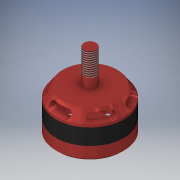
# Autodesk Inventor part: Motor
Saved by Autodesk Inventor 2019.3 (Build 233278000, 278)
## iProperties
Created: 2019-02-12
Part Number: Motor
Material: Aluminum 6061
Document SubType Name: Modeling
Designer: JMoll
Density: 2.7 g/cm^3
Appearance: Aluminum - Polished(1)
Author: JMoll
Autodesk Inventor part; units mm, degrees
sketch "Sketch1" plane through (0, 0, 0) normal (0, 0, 1) x (1, 0, 0)
  line L0 (0, 0) -> (0, 17.2)
  line L1 (0, 17.2) -> (11.25, 17.2)
  line L2 (11.25, 17.2) -> (14, 13.2)
  line L3 (14, 13.2) -> (14, 0)
  line L4 (14, 0) -> (0, 0)
  dimension "d0" = 17.2
  dimension "d1" = 28
  dimension "d2" = 22.5
  dimension "d3" = 13.2
  constraints: 10 end point, 2 perpendicular, 1 parallel, 1 vertical
  measures "d0" distance of L0.start L0.end
  measures "d1" diameter of L3 L0
  measures "d2" diameter of L1.end L0
  measures "d3" distance of L2.end L3.end
revolve "Revolution1" add sketch "Sketch1" angle 360 about axis through (0, 0, 0) along (0, 1, 0)
shell "Shell1" thickness 2.5 removed faces 0 ; own thickness 1 on faces at (1.3298, 17.2, -1.7114) ; own thickness 3.5 on faces at (2.651, 0, -3.8406)
sketch "Sketch2" plane through (0, 17.2, 0) normal (0, 1, 0) x (1, 0, 0)
  circle A0 centre (0, 0) radius 11.25 construction
  circle A1 centre (0, 0) radius 2.5
  dimension "d5" = 5
  constraints: 1 centre point, 1 coincident
  measures "d5" diameter of A1
extrude "Extrusion1" add sketch "Sketch2" along normal blind 14
thread "Thread1" size "M5x0.8" class "6g" standard "ANSI Metric M Profile" length 9.5
ref_plane "Work Plane1" through (0, 6.6, 14) normal (0, 0, 1) x (1, 0, 0)
sketch "Sketch3" plane through (0, 6.6, 14) normal (0, 0, 1) x (1, 0, 0)
  line L0 (-14, 6.6) -> (14, 6.6) construction
  line L1 (-11.25, 10.6) -> (11.25, 10.6) construction
  line L2 (0, 10.6) -> (0, 6.6) construction
  line L3 (-2.9, 8.1) -> (2.9, 8.1) construction
  line L4 (-2.9, 6.6) -> (2.9, 6.6)
  line L5 (2.9, 9.6) -> (-2.9, 9.6)
  arc A0 (-2.9, 9.6) -> (-2.9, 6.6) centre (-2.9, 8.1) ccw
  arc A1 (2.9, 6.6) -> (2.9, 9.6) centre (2.9, 8.1) ccw
  point P0 (0, -6.6)
  point P1 (0, 8.1)
  point P2 (0, 8.6)
  dimension "d13" = 5.8
  dimension "d16" = 1
  dimension "d17" = 4
  dimension "d18" = 13.2
  constraints: 10 end point, 5 midpoint, 4 point on circle, 4 tangent, 2 centre point, 1 horizontal, 1 parallel, 1 point on line
  measures "d13" distance of L3.start L3.end
  measures "d16" distance between parallel lines of L5 L1
  measures "d17" distance between parallel lines of L0 L1
  measures "d18" distance from line of point (0, -6.6) L0
extrude "Extrusion2" cut sketch "Sketch3" against normal through all
pattern_circular "Circular Pattern1" count 6 over 360 about axis through (0, 17.2, 0) along (0, 1, 0) of "Extrusion2"
ref_plane "Work Plane3" through (0, 12.1, 0) normal (0, -1, 0) x (1, 0, 0)
ref_plane "Work Plane2" through (0, 5.5, 0) normal (0, -1, 0) x (1, 0, 0)
split body "Split1" result two bodies by plane through (0, 5.5, 0) normal (0, -1, 0) first body at (2.651, 0.5, -3.8406)
split_face "Split2"
sketch "Sketch4" plane through (0, 0, 0) normal (0, -1, 0) x (1, 0, 0)
  circle A0 centre (0, 0) radius 14 projected
  line L0 (-1.71, 9) -> (1.71, 9) construction
  line L1 (-1.71, 6.5) -> (1.71, 6.5)
  line L2 (1.71, 11.5) -> (-1.71, 11.5)
  arc A1 (-1.71, 11.5) -> (-1.71, 6.5) centre (-1.71, 9) ccw
  arc A2 (1.71, 6.5) -> (1.71, 11.5) centre (1.71, 9) ccw
  line L3 (0, 14) -> (0, 11.5) construction
  point P0 (0, 9)
  point P1 (0, 6.5)
  dimension "d25" = 5
  dimension "d27" = 2.5
  dimension "d28" = 8.42
  constraints: 10 end point, 4 point on circle, 4 tangent, 4 vertical alignment, 3 midpoint, 2 centre point, 1 horizontal, 1 parallel, 1 vertical, 1 other
  measures "d25" distance between parallel lines of L2 L1
  measures "d27" distance of L3.start L3.end
extrude "Extrusion3" cut sketch "Sketch4" against normal blind 4 contours A1 L2 A2 L1 bodies 2
pattern_circular "Circular Pattern2" count 4 over 360 about axis through (0, -10, 0) along (0, 1, 0) of "Extrusion3" bodies 2
sketch "Sketch5" plane through (0, 0, 0) normal (0, -1, 0) x (1, 0, 0)
  circle A0 centre (0, 0) radius 14 projected
  circle A1 centre (0, 0) radius 4
  dimension "d34" = 8
  constraints: 1 centre point, 1 coincident
  measures "d34" diameter of A1
extrude "Extrusion4" cut sketch "Sketch5" against normal blind 2 contours A1 bodies 2
sketch "Sketch6" plane through (0, 0, 0) normal (0, 0, 1) x (1, 0, 0)
  line L0 (-11.5, 4) -> (-11.5, 0) construction
  line L1 (-11.5, 0) -> (-14, 0) construction
  line L2 (-14, 0) -> (-14, 5.5) construction
  line L3 (-11.5, 5.5) -> (-14, 5.5) construction
  line L4 (-11.5, 5.5) -> (-11.5, 4) construction
  line L5 (11.5, 0) -> (11.5, 4) construction
  line L6 (11.5, 4) -> (11.5, 5.5) construction
  line L7 (14, 5.5) -> (11.5, 5.5) construction
  line L8 (14, 5.5) -> (14, 0) construction
  line L9 (14, 0) -> (11.5, 0) construction
  line L10 (6.5, 3.5) -> (6.5, 0) projected
  line L11 (6.5, 0) -> (4, 0) projected
  line L12 (4, 0) -> (4, 2) projected
  line L13 (4, 2) -> (-4, 2) projected
  line L14 (-4, 2) -> (-4, 0) construction
  line L15 (-4, 0) -> (-6.5, 0) construction
  line L16 (-6.5, 0) -> (-6.5, 3.5) construction
  line L17 (-6.5, 3.5) -> (6.5, 3.5) projected
  line L18 (-14, 13.2) -> (-11.25, 17.2) construction
  line L19 (-11.25, 17.2) -> (-2.5, 17.2) construction
  line L20 (-2.5, 17.2) -> (-2.5, 31.2) construction
  line L21 (-2.5, 31.2) -> (2.5, 31.2) projected
  line L22 (2.5, 31.2) -> (2.5, 17.2) projected
  line L23 (2.5, 17.2) -> (11.25, 17.2) construction
  line L24 (11.25, 17.2) -> (14, 13.2) construction
  line L25 (11.5, 12.4235) -> (8.9037, 16.2) construction
  line L26 (8.9037, 16.2) -> (-8.9037, 16.2) construction
  line L27 (-8.9037, 16.2) -> (-11.5, 12.4235) construction
  line L28 (4, 2) -> (5, 0)
  line L29 (4, 0) -> (5, 0)
  line L30 (4, 0) -> (4, 2)
  line L31 (-11.5, 4) -> (-11.5, 0) construction
  line L32 (-11.5, 0) -> (-14, 0) construction
  line L33 (-14, 0) -> (-14, 5.5) construction
  line L34 (-11.5, 5.5) -> (-14, 5.5) construction
  line L35 (-11.5, 5.5) -> (-11.5, 4) construction
  line L36 (11.5, 0) -> (11.5, 4) construction
  line L37 (11.5, 4) -> (11.5, 5.5) construction
  line L38 (14, 5.5) -> (11.5, 5.5) construction
  line L39 (14, 5.5) -> (14, 0) construction
  line L40 (14, 0) -> (11.5, 0) construction
  line L41 (6.5, 3.5) -> (6.5, 0) projected
  line L42 (6.5, 0) -> (4, 0) projected
  line L43 (4, 0) -> (4, 2) projected
  line L44 (4, 2) -> (-4, 2) projected
  line L45 (-4, 2) -> (-4, 0) construction
  line L46 (-4, 0) -> (-6.5, 0) construction
  line L47 (-6.5, 0) -> (-6.5, 3.5) construction
  line L48 (-6.5, 3.5) -> (6.5, 3.5) projected
  line L49 (-14, 13.2) -> (-11.25, 17.2) construction
  line L50 (-11.25, 17.2) -> (-2.5, 17.2) construction
  line L51 (-2.5, 17.2) -> (-2.5, 31.2) construction
  line L52 (-2.5, 31.2) -> (2.5, 31.2) projected
  line L53 (2.5, 31.2) -> (2.5, 17.2) projected
  line L54 (2.5, 17.2) -> (11.25, 17.2) construction
  line L55 (11.25, 17.2) -> (14, 13.2) construction
  line L56 (11.5, 12.4235) -> (8.9037, 16.2) construction
  line L57 (8.9037, 16.2) -> (-8.9037, 16.2) construction
  line L58 (-8.9037, 16.2) -> (-11.5, 12.4235) construction
  line L59 (0, -6.24) -> (0, 37.44) projected
  line L60 (-14, 5.5) -> (-14, 12.1) projected
  line L61 (-14, 12.1) -> (-14, 13.2) projected
  line L62 (14, 13.2) -> (14, 12.1) projected
  line L63 (14, 12.1) -> (14, 5.5) projected
  line L64 (11.5, 5.5) -> (11.5, 12.4235) projected
  line L65 (-11.5, 12.4235) -> (-11.5, 5.5) projected
  line L66 (-14, 5.5) -> (-14, 12.1) projected
  line L67 (-14, 12.1) -> (-14, 13.2) projected
  line L68 (14, 13.2) -> (14, 12.1) projected
  line L69 (14, 12.1) -> (14, 5.5) projected
  line L70 (11.5, 5.5) -> (11.5, 12.4235) projected
  line L71 (-11.5, 12.4235) -> (-11.5, 5.5) projected
  point P0 (0, 0)
  dimension "d37" = 1
  constraints: 6 end point, 1 collinear, 1 perpendicular, 1 point on line
  measures "d37" distance from line of L12 L28.end
revolve "Revolution2" cut sketch "Sketch6" angle 360 about axis through (0, -10, 0) along (0, 1, 0) bodies 2 contours L11 L12 L28
sketch "Sketch7" plane through (0, 0, 0) normal (0, -1, 0) x (1, 0, 0)
  circle A0 centre (0, 0) radius 5 projected
  circle A1 centre (0, 0) radius 14 projected
  circle A2 centre (6.7175, 6.7175) radius 1.25
  line L0 (9.8995, 9.8995) -> (-9.8995, -9.8995) construction
  line L1 (-9.8995, 9.8995) -> (9.8995, -9.8995) construction
  line L2 (0, -14) -> (0, 14) construction
  circle A3 centre (-5.6569, 5.6569) radius 1.25
  circle A4 centre (5.6569, -5.6569) radius 1.25
  circle A5 centre (-6.7175, -6.7175) radius 1.25
  dimension "d40" = 90
  dimension "d41" = 45
  dimension "d42" = 4.5
  dimension "d43" = 2.5
  dimension "d44" = 2.5
  dimension "d45" = 6
  constraints: 6 end point, 6 point on circle, 4 centre point, 3 midpoint, 2 coincident, 2 point on line, 2 symmetric about line, 1 vertical, 2 other
  measures "d40" angle of L1 L0
  measures "d41" angle of L2 L1
  measures "d42" distance of L0.start A2.centre
  measures "d43" diameter of A2
  measures "d44" diameter of A3
  measures "d45" distance of L1.start A3.centre
ref_plane "Work Plane4" through (0, 0, -14) normal (0, 0, 1) x (1, 0, 0)
chamfer "Chamfer1" distance 1 angle 45 1 edges at (-14, 0, 0)
sketch "Sketch8" plane through (0, 0, -14) normal (0, 0, 1) x (1, 0, 0)
  line L0 (2.75, 2.75) -> (-2.75, 2.75) construction
  line L1 (2.75, 1) -> (-2.75, 1)
  line L2 (-2.75, 4.5) -> (2.75, 4.5)
  arc A0 (2.75, 1) -> (2.75, 4.5) centre (2.75, 2.75) ccw
  arc A1 (-2.75, 4.5) -> (-2.75, 1) centre (-2.75, 2.75) ccw
  line L3 (-14, 1) -> (14, 1) projected
  point P0 (0, 0)
  point P1 (0, 2.75)
  point P2 (0, 4.5)
  point P3 (0, 1)
  dimension "d52" = 9
  dimension "d53" = 3.5
  constraints: 8 end point, 4 midpoint, 4 point on circle, 4 tangent, 3 vertical alignment, 2 centre point, 1 horizontal, 1 parallel
  measures "d53" distance between parallel lines of L1 L2
extrude "Extrusion6" cut sketch "Sketch8" along normal up to surface round surface about axis through (0, 6.6, 0) along (0, -1, 0) radius 11.5 far side no bodies 2
hole "Hole1" at (6.7175, 0, 6.7175) at (5.6569, 0, -5.6569) at (-6.7175, 0, -6.7175) at (-5.6569, 0, 5.6569) direction (0, 1, 0) diameter 2.459 end through all bodies 2 thread size "M3x0.5" class "6H" standard "ISO Metric profile"
